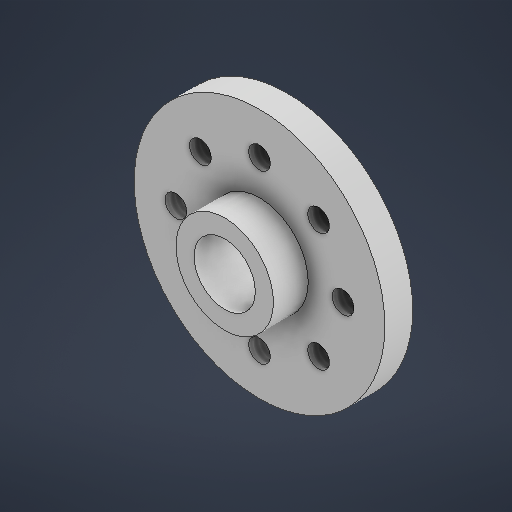
# Autodesk Inventor part: STS3032_Horn
Saved by Autodesk Inventor 2026 (Build 300175050, 175E)
## iProperties
Created: 2026-07-07
Part Number: STS3032_Horn
Material: 一般
Document SubType Name: Modeling
Designer: hanaj
Density: 1 g/cm^3
Appearance: 既定
Author: hanaj
Autodesk Inventor part; units mm, degrees
ref_plane "YZ Plane" through (0, 0, 0) normal (1, 0, 0) x (0, 1, 0)
ref_plane "XZ Plane" through (0, 0, 0) normal (0, 1, 0) x (-1, 0, 0)
ref_plane "XY Plane" through (0, 0, 0) normal (0, 0, 1) x (1, 0, 0)
sketch "スケッチ1" plane through (0, 0, 0) normal (0, 0, 1) x (1, 0, 0)
  circle A0 centre (0, 0) radius 9
  dimension "d0" = 18
  constraints: 1 centre point, 1 coincident
  measures "d0" diameter of A0
extrude "押し出し1" add sketch "スケッチ1" along normal blind 2
sketch "スケッチ2" plane through (0, 0, 2) normal (0, 0, 1) x (1, 0, 0)
  circle A0 centre (0, 0) radius 3.5
  dimension "d3" = 7
  constraints: 1 centre point, 1 coincident
  measures "d3" diameter of A0
extrude "押し出し2" add sketch "スケッチ2" along normal blind 2.5
sketch "スケッチ3" plane through (0, 0, 4.5) normal (0, 0, 1) x (1, 0, 0)
  circle A0 centre (0, 0) radius 2.2
  dimension "d6" = 4.4
  constraints: 1 centre point, 1 coincident
  measures "d6" diameter of A0
extrude "押し出し3" cut sketch "スケッチ3" against normal blind 3.3
sketch "スケッチ4" plane through (0, 0, 1.2) normal (0, 0, 1) x (1, 0, 0)
  circle A0 centre (0, 0) radius 2.2 projected
  circle A1 centre (0, 0) radius 1.15
  dimension "d9" = 2.3
  constraints: 1 centre point, 1 coincident
  measures "d9" diameter of A1
extrude "押し出し4" cut sketch "スケッチ4" against normal through all contours A1
sketch "スケッチ5" plane through (0, 0, 0) normal (0, 0, -1) x (-1, 0, 0)
  circle A0 centre (0, 0) radius 6 construction
  line L0 (0, -11.2961) -> (0, 11.2961) construction
  line L1 (-11.4539, 0) -> (11.4539, 0) construction
  point P0 (0, 6)
  point P1 (-4.2426, 4.2426)
  point P2 (-6, 0)
  point P3 (-4.2426, -4.2426)
  point P4 (0, -6)
  point P5 (4.2426, -4.2426)
  point P6 (6, 0)
  point P7 (4.2426, 4.2426)
  dimension "d12" = 12
  dimension "d15" = 360
  constraints: 4 end point, 2 midpoint, 1 coincident, 1 perpendicular, 1 point on line, 1 vertical, 1 vertical alignment, 11 other
hole "穴1" at (0, 6, 0) at (4.2426, 4.2426, 0) at (6, 0, 0) at (4.2426, -4.2426, 0) at (0, -6, 0) at (-4.2426, -4.2426, 0) at (-6, 0, 0) at (-4.2426, 4.2426, 0) direction (0, 0, 1) diameter 1.567 end through all thread size "M2x0.4" class "6H" standard "ISO Metric profile"
